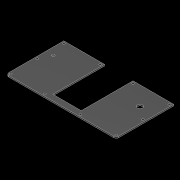
# Autodesk Inventor part: TopPlate
Saved by Autodesk Inventor 2021 (Build 250183000, 183)
## iProperties
Created: 2020-10-23
Part Number: TopPlate
Material: Nylon 6/6
Document SubType Name: Modeling
Designer: Esketitttttt
Density: 1.13 g/cm^3
Appearance: Smooth - Black
Mass: 11.4349 g
Surface Area: 136.96 cm^2
Volume: 10.1194 cm^3
Author: Esketitttttt
Autodesk Inventor part; units mm, degrees
ref_plane "YZ Plane" through (0, 0, 0) normal (1, 0, 0) x (0, 1, 0)
ref_plane "XZ Plane" through (0, 0, 0) normal (0, 1, 0) x (-1, 0, 0)
ref_plane "XY Plane" through (0, 0, 0) normal (0, 0, 1) x (1, 0, 0)
sketch "Sketch1" plane through (0, 0, 0) normal (0, 1, 0) x (-1, 0, 0)
  circle A0 centre (39.5667, 2.54) radius 1.016 construction
  circle A1 centre (35.24, -78.62) radius 1.0938 construction
  circle A2 centre (-56.4602, -0.58) radius 1.016 construction
  circle A3 centre (77.06, -78.62) radius 1.016 construction
  circle A4 centre (-1.4667, 2.54) radius 1.016 construction
  circle A5 centre (75.2, 2.54) radius 1.016 construction
  circle A6 centre (-2.54, -78.62) radius 1.016 construction
  circle A7 centre (-42.5, -78.62) radius 1.016 construction
  circle A8 centre (75.2, -40.58) radius 1.016 construction
  circle A9 centre (-42.5, 2.54) radius 1.016 construction
  line L0 (77.74, 5.08) -> (77.74, -44.73) construction
  line L1 (77.74, 5.08) -> (-45.04, 5.08) construction
  line L2 (-45.04, 5.08) -> (-45.04, -81.16) construction
  line L3 (-45.04, -81.16) -> (0, -81.16) construction
  line L4 (0, -76.08) -> (0, -81.16) construction
  line L5 (0, -76.08) -> (-39.96, -76.08) construction
  line L6 (-39.96, -76.08) -> (-39.96, 0) construction
  line L7 (-39.96, 0) -> (72.66, 0) construction
  line L8 (72.66, 0) -> (72.66, -76.08) construction
  line L9 (72.66, -76.08) -> (32.7, -76.08) construction
  line L10 (32.7, -76.08) -> (32.7, 0) construction
  line L11 (0, -76.08) -> (-39.96, -76.08) construction
  line L12 (-39.96, -76.08) -> (-39.96, 0) construction
  line L13 (-39.96, 0) -> (0, 0) construction
  line L14 (0, 0) -> (0, -76.08) construction
  line L15 (32.7, -76.08) -> (72.66, -76.08) construction
  line L16 (72.66, -76.08) -> (72.66, 0) construction
  line L17 (72.66, 0) -> (32.7, 0) construction
  line L18 (32.7, 0) -> (32.7, -76.08) construction
  line L19 (32.7, 0) -> (0, 0) construction
  line L20 (0, 0) -> (0, -2.4299) construction
  line L21 (0, -2.4299) -> (32.7, -2.4299) construction
  line L22 (32.7, -2.4299) -> (32.7, 0) construction
  circle A10 centre (-2.54, -78.62) radius 1.0922 construction
  circle A11 centre (-42.5, -78.62) radius 1.0922 construction
  circle A12 centre (-56.4602, -0.58) radius 1.0922 construction
  circle A13 centre (-42.5, 2.54) radius 1.0922 construction
  circle A14 centre (-1.4667, 2.54) radius 1.0924 construction
  circle A15 centre (39.5667, 2.54) radius 1.0924 construction
  circle A16 centre (75.2, 2.54) radius 1.0924 construction
  circle A17 centre (75.2, -40.58) radius 1.0924 construction
  circle A18 centre (77.06, -78.62) radius 1.0924 construction
  circle A19 centre (35.24, -78.62) radius 1.0938 construction
  line L23 (77.06, -78.62) -> (74.52, -78.62) construction
  line L24 (74.52, -78.62) -> (71.345, -78.62) construction
  circle A20 centre (71.345, -40.74) radius 1.5875
  line L25 (-56.4602, -0.58) -> (-2.54, -78.62) construction
  circle A21 centre (-29.5001, -39.6) radius 3
  circle A22 centre (37.7067, 2.54) radius 1.2192 construction
  circle A23 centre (35.24, -78.62) radius 1.0938 construction
  circle A24 centre (-44.36, -40.58) radius 1.0922 construction
  circle A25 centre (77.06, -78.62) radius 1.0922 construction
  circle A26 centre (-3.3267, 2.54) radius 1.2192 construction
  circle A27 centre (77.06, 2.54) radius 1.0922 construction
  circle A28 centre (-2.54, -78.62) radius 1.016 construction
  circle A29 centre (-44.36, -78.62) radius 1.016 construction
  circle A30 centre (77.06, -40.58) radius 1.0922 construction
  circle A31 centre (-44.36, 2.54) radius 1.0922 construction
  line L26 (32.7, -81.16) -> (79.6, -81.16) construction
  line L27 (79.6, 5.08) -> (79.6, -81.16) construction
  line L28 (79.6, 5.08) -> (-46.9, 5.08) construction
  line L29 (-46.9, 5.08) -> (-46.9, -81.16) construction
  line L30 (-46.9, -81.16) -> (0, -81.16) construction
  line L31 (0, -76.08) -> (0, -81.16) construction
  line L32 (0, -76.08) -> (-41.82, -76.08) construction
  line L33 (-41.82, -76.08) -> (-41.82, 0) construction
  line L34 (-41.82, 0) -> (74.52, 0) construction
  line L35 (74.52, 0) -> (74.52, -76.08) construction
  line L36 (74.52, -76.08) -> (32.7, -76.08) construction
  line L37 (32.7, -76.08) -> (32.7, -81.16) construction
  line L38 (79.6, 5.08) -> (-46.9, 5.08)
  line L39 (-46.9, 5.08) -> (-46.9, -61.16)
  line L40 (-46.9, -61.16) -> (0, -61.16)
  line L41 (0, -61.16) -> (0, -56.08)
  line L42 (0, -56.08) -> (-41.82, -56.08)
  line L43 (-41.82, -56.08) -> (-41.82, 0)
  line L44 (-41.82, 0) -> (74.52, 0)
  line L45 (74.52, 0) -> (74.52, -56.08)
  line L46 (74.52, -56.08) -> (32.7, -56.08)
  line L47 (32.7, -56.08) -> (32.7, -61.16)
  line L48 (32.7, -61.16) -> (79.6, -61.16)
  line L49 (79.6, -61.16) -> (79.6, 5.08)
  line L50 (-41.82, 0) -> (74.52, 0)
  line L51 (79.6, 5.08) -> (79.6, -61.16)
  line L52 (74.52, 0) -> (79.6, 5.08) construction
  circle A32 centre (77.06, 2.54) radius 1.2192
  line L53 (74.52, 0) -> (74.52, -56.08)
  line L54 (74.52, -56.08) -> (79.6, -61.16) construction
  line L55 (32.7, -61.16) -> (79.6, -61.16)
  line L56 (32.7, -61.16) -> (37.78, -56.08) construction
  line L57 (74.52, -56.08) -> (32.7, -56.08)
  line L58 (0, -61.16) -> (0, -56.08)
  line L59 (0, -61.16) -> (-5.08, -56.08) construction
  line L60 (0, -56.08) -> (-41.82, -56.08)
  line L61 (79.6, 5.08) -> (-46.9, 5.08)
  line L62 (-46.9, 5.08) -> (-41.82, 0) construction
  line L63 (-41.82, -56.08) -> (-41.82, 0)
  line L64 (-46.9, 5.08) -> (-46.9, -61.16)
  line L65 (-41.82, -56.08) -> (-46.9, -61.16) construction
  circle A33 centre (77.06, -58.62) radius 1.2192
  circle A34 centre (35.24, -58.62) radius 1.2192
  circle A35 centre (-2.54, -58.62) radius 1.2192
  circle A36 centre (-44.36, -58.62) radius 1.2192
  circle A37 centre (-44.36, 2.54) radius 1.2192
  circle A38 centre (-3.3267, 2.54) radius 1.2192
  circle A39 centre (37.7067, 2.54) radius 1.2192
  circle A40 centre (77.06, -28.04) radius 1.2192
  circle A41 centre (-44.36, -28.04) radius 1.2192
  line L66 (32.7, -56.08) -> (32.7, -2.4299)
  line L67 (0, -2.4299) -> (32.7, -2.4299)
  line L68 (0, -2.4299) -> (0, -56.08)
  point P0 (32.7, -2.4299)
  point P1 (-1.86, -76.08)
  dimension "d0" = 2.4299
  dimension "d1" = 2.1844
  dimension "d2" = 2.1844
  dimension "d5" = 3.175
  dimension "d7" = 3.175
  dimension "d10" = 6
  dimension "d13" = 2.1877
  dimension "d14" = 2.1877
  dimension "d15" = 2.1844
  dimension "d16" = 2.1844
  dimension "d17" = 2.1844
  dimension "d18" = 2.4384
  dimension "d19" = 2.4384
  dimension "d20" = 2.1844
  dimension "d21" = 2.1844
  dimension "d24" = 5.08
  dimension "d29" = 86.24
  dimension "d30" = 5.08
  dimension "d31" = 5.08
  dimension "d32" = 5.08
  dimension "d33" = 5.08
  dimension "d34" = 126.5
  dimension "d35" = 5.08
  dimension "d36" = 5.08
  dimension "d37" = 5.08
  dimension "d38" = 5.08
  dimension "d39" = 2.54
  dimension "d40" = 2.54
  dimension "d41" = 2.54
  dimension "d42" = 2.54
  dimension "d56" = 2.4384
  dimension "d57" = 2.4384
  dimension "d58" = 2.4384
  dimension "d59" = 2.4384
  dimension "d60" = 2.4384
  dimension "d61" = 2.4384
  dimension "d62" = 41.0333
  dimension "d63" = 30.58
  dimension "d64" = 30.58
  dimension "d65" = 61.16
  dimension "d69" = 20.42
  dimension "d70" = 21.56
  constraints: 134 end point, 42 centre point, 14 horizontal, 12 parallel, 10 coincident, 8 perpendicular, 8 vertical, 7 midpoint, 3 point on line, 2 collinear, 25 other
  measures "d0" distance of L20.end L19.end
  measures "d1" diameter of A10
  measures "d2" diameter of A11
  measures "d5" distance of L23.end L24.end
  measures "d7" diameter of A20
  measures "d10" diameter of A21
  measures "d13" diameter of A1
  measures "d14" diameter of A23
  measures "d15" diameter of A25
  measures "d16" diameter of A30
  measures "d17" diameter of A27
  measures "d18" diameter of A22
  measures "d19" diameter of A26
  measures "d20" diameter of A31
  measures "d21" diameter of A24
  measures "d24" distance between parallel lines of L27 L35
  measures "d29" distance of L29.start L29.end
  measures "d30" distance of L4.start L3.end
  measures "d31" distance of L37.start L37.end
  measures "d32" distance between parallel lines of L33 L29
  measures "d33" distance between parallel lines of L1 L7
  measures "d34" distance of L28.start L29.start
  measures "d35" distance between parallel lines of L3 L5
  measures "d36" distance between parallel lines of L26 L15
  measures "d37" distance from line of L1 L17.end
  measures "d38" distance from line of L1 point (0, 0)
  measures "d39" distance from line of L5 A6.centre
  measures "d40" distance from line of L29 A29.centre
  measures "d41" distance from line of L9 A1.centre
  measures "d42" distance from line of L26 A3.centre
  measures "d56" diameter of A32
  measures "d57" diameter of A33
  measures "d58" diameter of A34
  measures "d59" diameter of A35
  measures "d60" diameter of A36
  measures "d61" diameter of A37
  measures "d62" distance of A37.centre A38.centre
  measures "d63" distance of A32.centre A40.centre
  measures "d64" distance of A37.centre A41.centre
  measures "d65" distance of A36.centre A37.centre
  measures "d69" distance from line of L55 A20.centre
  measures "d70" distance from line of L40 A21.centre
extrude "Extrusion3" add sketch "Sketch1" along normal blind 1.5875
fillet "Fillet2" radius 3.175 2 edges at (-79.6, 0.7937, 5.08) (46.9, 0.7937, 5.08)
chamfer "Chamfer1" distance 0.7937 angle 45 1 edges at (-16.35, 1.5875, -2.4299)
equation "\"d63\" = 0.5 * d65"
equation "\"d64\" = 0.5 * d65"
body "Solid3"
